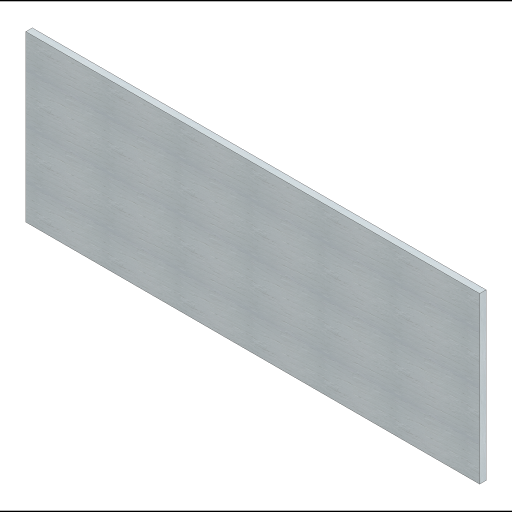
# Autodesk Inventor part: Wind Tunnel Settling Chamber Side As-Built
Saved by Autodesk Inventor 2023 (Build 270158000, 158)
## iProperties
Created: 2023-01-19
Part Number: Wind Tunnel Settling Chamber Side As-Built
Material: Wood (Oak)
Document SubType Name: Modeling
Designer: kamer
Density: 0.76 g/cm^3
Appearance: Wood - Painted White
Author: kamer
Autodesk Inventor part; units mm, degrees
ref_plane "YZ Plane" through (0, 0, 0) normal (1, 0, 0) x (0, 1, 0)
ref_plane "XZ Plane" through (0, 0, 0) normal (0, 1, 0) x (-1, 0, 0)
ref_plane "XY Plane" through (0, 0, 0) normal (0, 0, 1) x (1, 0, 0)
sketch "Sketch1" plane through (0, 0, 0) normal (0, 0, 1) x (1, 0, 0)
  line L0 (0, 0) -> (838.2, 0)
  line L1 (838.2, 0) -> (838.2, 304.8)
  line L2 (838.2, 304.8) -> (0, 304.8)
  line L3 (0, 304.8) -> (0, 0)
  dimension "d0" = 304.8
  dimension "d1" = 838.2
  constraints: 8 end point, 2 parallel, 1 horizontal, 1 perpendicular
  measures "d0" distance of L0.end L1.end
  measures "d1" distance of L1.end L2.end
extrude "Extrusion1" add sketch "Sketch1" along normal blind 11.938
body "Solid1"
